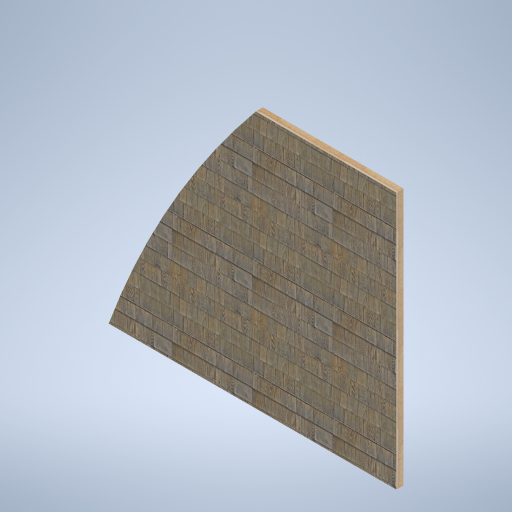
# Autodesk Inventor part: front_wall_block02
Saved by Autodesk Inventor 2024.2 (Build 282272000, 272)
## iProperties
Created: 2024-05-21
Part Number: front_wall_block02
Material: Wood (Maple)
Document SubType Name: Modeling
Designer: LOSTER_1
Density: 0.67 g/cm^3
Appearance: Natural Maple - Glossy Dark Tint
Author: LOSTER_1
Autodesk Inventor part; units mm, degrees
ref_plane "YZ Plane" through (0, 0, 0) normal (1, 0, 0) x (0, 1, 0)
ref_plane "XZ Plane" through (0, 0, 0) normal (0, 1, 0) x (-1, 0, 0)
ref_plane "XY Plane" through (0, 0, 0) normal (0, 0, 1) x (1, 0, 0)
sketch "Sketch1" plane through (0, 0, 0) normal (0, 0, 1) x (1, 0, 0)
  line L0 (-2952.1677, 2077.9155) -> (-1351.8191, 2077.9155)
  arc A0 (-2952.1677, 2077.9155) -> (-4628.6725, -853.7094) centre (4765.7133, -4280.8825) ccw
  line L1 (-1351.8191, 2077.9155) -> (-1351.8191, -853.7094)
  line L2 (-1351.8191, -853.7094) -> (-4628.6725, -853.7094)
  constraints: 6 end point, 2 point on circle, 1 centre point
extrude "Extrusion1" add sketch "Sketch1" along normal blind 80
body "Solid1"
